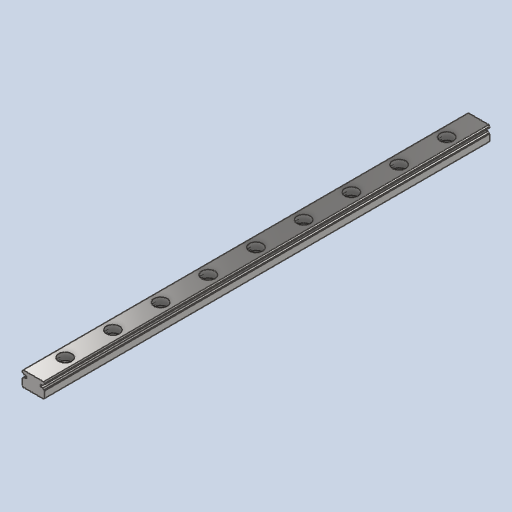
# Autodesk Inventor part: SSE2BLZ8-140_r1
Saved by Autodesk Inventor 2023 (Build 270158000, 158)
## iProperties
Category: PARTsolutions
Company: MISUMI
Created: 2024-12-13
Part Number: SSE2BLZ8-140_r1
Material: ステンレス鋼
Catalog Web Link: www.cadenas.de
Description: SEBSZ, SE2BSZ, SSEBSZ, SSEBSZ-MX, SSE2BSZ, SSE2BSLZ-MX, SEBSLZ, SE2BSLZ, SSEBSLZ, SSEBSZ-MX, SSE2BSLZ, SSE2BSLZ-MX_rail-Miniature Linear Guides - Short Blocks, Light Preload
Vendor: MISUMI
Document SubType Name: Modeling
Designer: psAdmin
Manufacturer: MISUMI
Mass: 30.7859 g
Surface Area: 41.5693 cm^2
Volume: 3.84823 cm^3
Density: 8 g/cm^3
Appearance: 半つや出し
PSOL_IDENT_0: {$CADENAS_DATA/23d-libs/misumi/metric/06_linear_guides/sebsz_series/sebsz_rail.prj},317 {VTYP=3D},{N
PSOL_IDENT_1: B=SSE2BLZ8-140_r1},{LINA=SSE2BLZ8-140},{NN=SEBSZ, SE2BSZ, SSEBSZ, SSEBSZ-MX, SSE2BSZ, SSE2BSLZ-MX, S
PSOL_IDENT_2: EBSLZ, SE2BSLZ, SSEBSLZ, SSEBSZ-MX, SSE2BSLZ, SSE2BSLZ-MX_rail},{DATE=16.02.2022 05:47:06},{GEOMDATE=
PSOL_IDENT_3: 21.01.2022 05:00:42},{VERSION=},{LINEID=90},{WBVAR=TS,LT,NOB,L,MAT,ST,MX,ALT1,ALT2,ALT4},{WBNUMERIC=
PSOL_IDENT_4: L}  {NB=SSE2BLZ8-140_r1},{LINA=SSE2BLZ8-140},{KT=DUMMY},{PN=SSE2BLZ8-140},{RT=B},{TS=},{TS1=  '','Ad
PSOL_IDENT_5: vanced','V','Precision'  },{TYPE=SSE2BLZ},{H=8},{LT=Configurable},{LTALG='Selectable','Selectable','
PSOL_IDENT_6: Configurable','Configurable'},{NOB=2},{L=140},{MAT=S},{ST=S},{MX=},{MXALG= '','w/o MX(Lubrication un
PSOL_IDENT_7: it)' },{ALT3=},{HARD=56HRC~},{W=17},{L1=19.6},{B=12},{C=8},{SLL=M2x2.5},{L2=9.6},{K=6.5},{CBB=0.3},{
PSOL_IDENT_8: W1=7},{W2=5.0},{H1=4.7},{CAA=0.3},{DD1DD2HH=2.4x4.2x2.3},{F=15},{G=10},{DD1=2.400},{DD2=4.200},{HH=2
PSOL_IDENT_9: .300},{ALT1=},{MC=M3},{MC1=3.0},{ALT2=},{ALT2L=0.0},{ALT2N=0},{M=9},{S1=M2},{LL1=2.5},{S2=M3},{NT=0.
PSOL_IDENT_10: 0},{LL=L},{L0=[56:69/1],[71:84/1],[86:99/1],[101:114/1],[116:129/1],[131:144/1],[146:159/1],[161:174
PSOL_IDENT_11: /1],[176:189/1],[191:204/1],[206:219/1],[221:234/1],[236:249/1],[251:264/1],[266:279/1],[281:294/1],
PSOL_IDENT_12: [296:309/1]},{REC1=   '','N/A'    },{CL=0.000},{BCR=    '','w/o Surface Treatment','-BCR','with BCR
PSOL_IDENT_13: (Surface Treatment)'    },{ST1='S', 'w/o Surface Treatment','R','Low Temperature Black Chrome Platin
PSOL_IDENT_14: g'},{MAT2='','Carbon Steel','S','Stainless Steel'},{LSC=6.0},{MS=2.0},{NL=35.000},{ALT4=},{ALT4ALG= ''
PSOL_IDENT_15: ,'N/A' },{CA1=0.3},{CA2=0.3},{VA1=1.5},{HA1=1.3},{HA2=7.4140},{WA1=1.6677},{WA2=0.7},{RA1=1.75},{POI
PSOL_IDENT_16: A1=0.1140},{NA1=8}
NB: SSE2BLZ8-140_r1
NN: SEBSZ, SE2BSZ, SSEBSZ, SSEBSZ-MX, SSE2BSZ, SSE2BSLZ-MX, SEBSLZ, SE2BSLZ, SSEBSLZ, SSEBSZ-MX, SSE2BSLZ, SSE2BSLZ-MX_rail
NT: Miniature Linear Guides - Short Blocks, Light Preload
NBSYN: $PN._r1
LINA: SSE2BLZ8-140
CATALOG: Misumi
PN: SSE2BLZ8-140
TS: Advanced
H: 8
LT: Configurable
NOB: 2
L: 140
MAT: Stainless Steel
ST: w/o Surface Treatment
MX: w/o MX(Lubrication unit)
W: 17
L1: 19.6
B: 12
C: 8
SLL: M2x2.5
L2: 9.6
K: 6.5
CBB: 0.3
W1: 7
W2: 5
H1: 4.7
CAA: 0.3
DD1DD2HH: 2.4x4.2x2.3
F: 15
G: 10
DD1: 2.4
DD2: 4.2
HH: 2.3
ALT1: w/o MC (Tapped Holes)
MC: M3
MC1: 3
ALT2: N/A
ALT2L: 0
ALT2N: 0
S1: M2
LL1: 2.5
S2: M3
CL: 0
LSC: 6
MS: 2
ALT4: N/A
CA1: 0.3
CA2: 0.3
VA1: 1.5
HA1: 1.3
HA2: 7.414
WA1: 1.6677
WA2: 0.7
RA1: 1.75
POIA1: 0.114
SUPPLIER: MISUMI
ARTICLENO: SSE2BLZ8-140_r1
BOMINFO: SSE2BLZ8-140
CREATOR: CADENAS GmbH
Title: SSE2BLZ8-140
Author: Cadenas PARTsolutions
Comments: Miniature Linear Guides - Short Blocks, Light Preload
Autodesk Inventor part; units mm, degrees
sketch "Sketch_12" plane through (0, 0, 0) normal (0, 0, 1) x (1, 0, 0)
  line L0 (-3.5, 4.4) -> (-3.5, 4.0339)
  line L1 (-3.5, 4.0339) -> (-3.2695, 3.9008)
  arc A0 (-2.9324, 3.55) -> (-3.2695, 3.9008) centre (-3.707, 3.143) ccw
  line L2 (-2.9324, 3.55) -> (-2.2, 3.55)
  line L3 (-2.2, 3.55) -> (-2.2, 2.85)
  line L4 (-2.2, 2.85) -> (-2.9324, 2.85)
  arc A1 (-3.2695, 2.4992) -> (-2.9324, 2.85) centre (-3.707, 3.257) ccw
  line L5 (-3.2695, 2.4992) -> (-3.5, 2.3662)
  line L6 (-3.5, 2.3662) -> (-3.5, 0.3)
  line L7 (-3.5, 0.3) -> (-3.2, 0)
  line L8 (-3.2, 0) -> (3.2, 0)
  line L9 (3.2, 0) -> (3.5, 0.3)
  line L10 (3.5, 0.3) -> (3.5, 2.3662)
  line L11 (3.5, 2.3662) -> (3.2695, 2.4992)
  arc A2 (2.9324, 2.85) -> (3.2695, 2.4992) centre (3.707, 3.257) ccw
  line L12 (2.9324, 2.85) -> (2.2, 2.85)
  line L13 (2.2, 2.85) -> (2.2, 3.55)
  line L14 (2.2, 3.55) -> (2.9324, 3.55)
  arc A3 (3.2695, 3.9008) -> (2.9324, 3.55) centre (3.707, 3.143) ccw
  line L15 (3.2695, 3.9008) -> (3.5, 4.0339)
  line L16 (3.5, 4.0339) -> (3.5, 4.4)
  line L17 (3.5, 4.4) -> (3.2, 4.7)
  line L18 (3.2, 4.7) -> (-3.2, 4.7)
  line L19 (-3.2, 4.7) -> (-3.5, 4.4)
  constraints: 40 end point, 8 point on circle, 4 centre point
extrude "Extrusion1" add sketch "Sketch_12" along normal mid plane 140
sketch "Sketch2" plane through (-3.2, 4.7, 70) normal (0, 1, 0) x (1, 0, 0)
  point P0 (3.2, 130)
hole "Hole1" at (0, 4.7, -60) direction (0, -1, 0) diameter 2.4 depth 4.7 counterbore diameter 4.2 counterbore depth 2.3
pattern_linear "Rectangular Pattern1" count 9 spacing 15 along (0, 0, 1) of "Hole1"
ref_plane "to_block_XY" through (0, 4.7, 35) normal (0, 0, -1) x (1, 0, 0)
ref_plane "to_block_YZ" through (0, 4.7, 35) normal (1, 0, 0) x (0, -1, 0)
ref_plane "to_block_ZX" through (0, 4.7, 35) normal (0, -1, 0) x (0, 0, -1)
ref_plane "to_block_2_XY" through (0, 4.7, -35) normal (0, 0, -1) x (1, 0, 0)
ref_plane "to_block_2_YZ" through (0, 4.7, -35) normal (1, 0, 0) x (0, -1, 0)
ref_plane "to_block_2_ZX" through (0, 4.7, -35) normal (0, -1, 0) x (0, 0, -1)
ref_plane "to_bolt_1_XY" through (0, 2.4, 60) normal (0, 1, 0) x (1, 0, 0)
ref_plane "to_bolt_1_YZ" through (0, 2.4, 60) normal (1, 0, 0) x (0, 0, -1)
ref_plane "to_bolt_1_ZX" through (0, 2.4, 60) normal (0, 0, -1) x (0, 1, 0)
ref_plane "to_bolt_2_XY" through (0, 2.4, 45) normal (0, 1, 0) x (1, 0, 0)
ref_plane "to_bolt_2_YZ" through (0, 2.4, 45) normal (1, 0, 0) x (0, 0, -1)
ref_plane "to_bolt_2_ZX" through (0, 2.4, 45) normal (0, 0, -1) x (0, 1, 0)
ref_plane "to_bolt_3_XY" through (0, 2.4, 30) normal (0, 1, 0) x (1, 0, 0)
ref_plane "to_bolt_3_YZ" through (0, 2.4, 30) normal (1, 0, 0) x (0, 0, -1)
ref_plane "to_bolt_3_ZX" through (0, 2.4, 30) normal (0, 0, -1) x (0, 1, 0)
ref_plane "to_bolt_4_XY" through (0, 2.4, 15) normal (0, 1, 0) x (1, 0, 0)
ref_plane "to_bolt_4_YZ" through (0, 2.4, 15) normal (1, 0, 0) x (0, 0, -1)
ref_plane "to_bolt_4_ZX" through (0, 2.4, 15) normal (0, 0, -1) x (0, 1, 0)
ref_plane "to_bolt_5_XY" through (0, 2.4, 0) normal (0, 1, 0) x (1, 0, 0)
ref_plane "to_bolt_5_YZ" through (0, 2.4, 0) normal (1, 0, 0) x (0, 0, -1)
ref_plane "to_bolt_5_ZX" through (0, 2.4, 0) normal (0, 0, -1) x (0, 1, 0)
ref_plane "to_bolt_6_XY" through (0, 2.4, -15) normal (0, 1, 0) x (1, 0, 0)
ref_plane "to_bolt_6_YZ" through (0, 2.4, -15) normal (1, 0, 0) x (0, 0, -1)
ref_plane "to_bolt_6_ZX" through (0, 2.4, -15) normal (0, 0, -1) x (0, 1, 0)
ref_plane "to_bolt_7_XY" through (0, 2.4, -30) normal (0, 1, 0) x (1, 0, 0)
ref_plane "to_bolt_7_YZ" through (0, 2.4, -30) normal (1, 0, 0) x (0, 0, -1)
ref_plane "to_bolt_7_ZX" through (0, 2.4, -30) normal (0, 0, -1) x (0, 1, 0)
ref_plane "to_bolt_8_XY" through (0, 2.4, -45) normal (0, 1, 0) x (1, 0, 0)
ref_plane "to_bolt_8_YZ" through (0, 2.4, -45) normal (1, 0, 0) x (0, 0, -1)
ref_plane "to_bolt_8_ZX" through (0, 2.4, -45) normal (0, 0, -1) x (0, 1, 0)
ref_plane "to_bolt_9_XY" through (0, 2.4, -60) normal (0, 1, 0) x (1, 0, 0)
ref_plane "to_bolt_9_YZ" through (0, 2.4, -60) normal (1, 0, 0) x (0, 0, -1)
ref_plane "to_bolt_9_ZX" through (0, 2.4, -60) normal (0, 0, -1) x (0, 1, 0)
body "Solid1"
